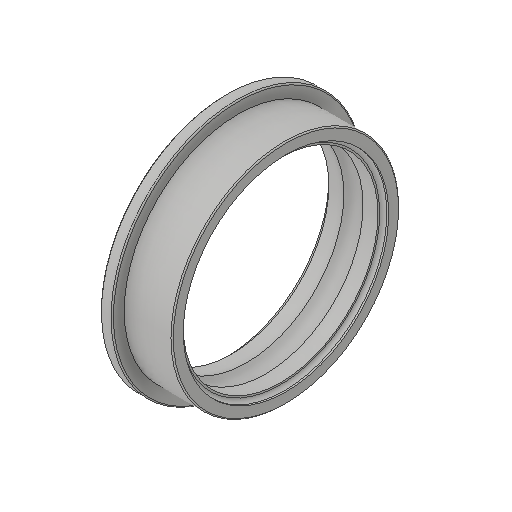
# Autodesk Inventor part: SKF_W 61800 R-2RS1_PART2
Saved by Autodesk Inventor 2022 (Build 260153000, 153)
## iProperties
Category: PARTsolutions
Company: SKF
Created: 2022-07-26
Part Number: SKF_W 61800 R-2RS1_PART2
Material: Generic
Catalog Web Link: www.cadenas.de
Description: -Deep groove ball bearings
Vendor: SKF
Document SubType Name: Modeling
Designer: psAdmin
Manufacturer: SKF
Mass: 6 g
Surface Area: 8.28117 cm^2
Volume: 0.405139 cm^3
Density: 1 g/cm^3
Appearance: PSOLRGB-175-175-175
PSOL_IDENT_0: {$CADENAS_DATA/23d-libs/skf/bearings_units_and_housings/ball_bearings/deep_groove_ball_bearings/bb1_
PSOL_IDENT_1: 001_101.prj},215 {VTYP=3D},{NB=SKF_W 61800 R-2RS1_PART2},{LINA=SKF_W 61800 R-2RS1_PART2},{NN=BB1_001
PSOL_IDENT_2: _101_PART2},{NOPRJ=TRUE},{DATE=08.07.2022 10:24:27},{GEOMDATE=04.07.2022 10:54:51},{VERSION=},{LINEI
PSOL_IDENT_3: D=22520},{WBVAR=},{WBNUMERIC=}  {NB=SKF_W 61800 R-2RS1_PART2},{LINA=SKF_W 61800 R-2RS1_PART2},{KT=DU
PSOL_IDENT_4: MMY},{DESIGNATION=W 61800 R-2RS1},{R12=0.30},{DD=10.000},{D=19.000},{B=5.000},{C=},{CX=},{CXX=1},{CA=
PSOL_IDENT_5: 1.000},{XXVARIANT=Flanged outer ring},{XXDESIGN=Single row stainless steel},{XXSEALING=Contact seal
PSOL_IDENT_6: on both sides},{DESIGN=dgbbwr2zs},{DESIGNIR=dgbbwr2zs},{VARIANT=Flanged outer ring},{DD1=12.74},{DD2=
PSOL_IDENT_7: 11.8},{DD2X=},{DD2A=11.80},{D1=16.26},{D1X=0.00},{D2=17.15},{D2A=17.15},{D3=21},{D3X=},{D3A=21.000},
PSOL_IDENT_8: {D4=},{HH=0.000},{BB=0.000},{BBX=},{BBA=0.000},{FF=},{R0MAX=0.000},{R0=0.000},{PITCH=14.50},{DW=2.38
PSOL_IDENT_9: 1},{DDAMIN=11.500},{DDAMAX=11.500},{DDBMIN=0.000},{DDBMAX=0.000},{DBMIN=0.000},{DAMAX=0.000},{BBAMIN=
PSOL_IDENT_10: 0.000},{CAMAX=0.000},{RAMAX=0.300},{LOAD1=1.480},{LOAD2=0.830},{LOAD3=0.036},{SPEED1=0},{SPEED2=2200
PSOL_IDENT_11: 0},{KR=0.020},{F0=14.800},{Z=10},{II=1},{MASS=0.006},{BEARING=W 61800 R-2RS1},{RING=},{HELP=1.370},{
PSOL_IDENT_12: HELP2=0.925},{DD1ALG=6.370},{YALG=6.370},{PITCH1=14.500},{DW1=2.381},{YALG1=8.130},{HALG1=1.370},{SH=
PSOL_IDENT_13: 5.900},{CU=0.524},{HALG=1.37},{B1=-2.82145},{SHIELDHELP=2},{D4A=0.000},{FFA=0.000},{RS1=},{HELP3=0}
NB: SKF_W 61800 R-2RS1_PART2
NT: Deep groove ball bearings
NBSYN: SKF_$DESIGNATION._PART2
LINA: SKF_W 61800 R-2RS1_PART2
CATALOG: SKF
DESIGNATION: W 61800 R-2RS1
R12: 0.3
DD: 10
D: 19
B: 5
XXVARIANT: Flanged outer ring
XXDESIGN: Single row stainless steel
XXSEALING: Contact seal on both sides
DD2: 11.8
D2: 17.15
LOAD1: 1.48
LOAD2: 0.83
LOAD3: 0.036
SPEED1: 0
SPEED2: 22000
BEARING: W 61800 R-2RS1
SUPPLIER: SKF
ARTICLENO: SKF_W 61800 R-2RS1_PART2
BOMINFO: SKF_W 61800 R-2RS1_PART2
CREATOR: CADENAS GmbH
Title: SKF_W 61800 R-2RS1_PART2
Author: Cadenas PARTsolutions
Comments: Deep groove ball bearings
Autodesk Inventor part; units mm, degrees
ref_plane "YZ Plane" through (0, 0, 0) normal (1, 0, 0) x (0, 1, 0)
ref_plane "XZ Plane" through (0, 0, 0) normal (0, 1, 0) x (-1, 0, 0)
ref_plane "XY Plane" through (0, 0, 0) normal (0, 0, 1) x (1, 0, 0)
sketch "Sketch_21" plane through (0, 0, 0) normal (0, 0, 1) x (1, 0, 0)
  line L0 (50, 0) -> (-50, 0)
  line L1 (0, 10.4) -> (0, 8.575)
  line L2 (0, 8.575) -> (0.15, 8.575)
  arc A0 (0.45, 8.275) -> (0.15, 8.575) centre (0.15, 8.275) ccw
  line L3 (0.45, 8.275) -> (0.45, 8.13)
  line L4 (0.45, 8.13) -> (1.6982, 8.13)
  arc A1 (3.3018, 8.13) -> (1.6982, 8.13) centre (2.5, 7.25) ccw
  line L5 (3.3018, 8.13) -> (4.55, 8.13)
  line L6 (4.55, 8.13) -> (4.55, 8.275)
  arc A2 (4.85, 8.575) -> (4.55, 8.275) centre (4.85, 8.275) ccw
  line L7 (4.85, 8.575) -> (5, 8.575)
  line L8 (5, 8.575) -> (5, 9.4)
  arc A3 (5, 9.4) -> (4.9, 9.5) centre (4.9, 9.4) ccw
  line L9 (4.9, 9.5) -> (1, 9.5)
  line L10 (1, 9.5) -> (1, 10.4)
  arc A4 (1, 10.4) -> (0.9, 10.5) centre (0.9, 10.4) ccw
  line L11 (0.9, 10.5) -> (0.1, 10.5)
  arc A5 (0.1, 10.5) -> (0, 10.4) centre (0.1, 10.4) ccw
  constraints: 24 end point, 12 point on circle, 6 centre point
revolve "Revolution1" add sketch "Sketch_21" angle 360 about axis through (50, 0, 0) along (1, 0, 0)
body "Solid1"
